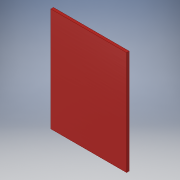
# Autodesk Inventor part: GBX_001.1-side-plate
Saved by Autodesk Inventor 2019 (Build 230136000, 136)
## iProperties
Created: 2019-08-15
Part Number: GBX_001.1-side-plate
Material: Generic
Document SubType Name: Modeling
Designer: Rene
Density: 1 g/cm^3
Appearance: Orange-Red
Author: Rene
Autodesk Inventor part; units mm, degrees
ref_plane "YZ Plane" through (0, 0, 0) normal (1, 0, 0) x (0, 1, 0)
ref_plane "XZ Plane" through (0, 0, 0) normal (0, 1, 0) x (-1, 0, 0)
ref_plane "XY Plane" through (0, 0, 0) normal (0, 0, 1) x (1, 0, 0)
sketch "Sketch1" plane through (0, 0, 0) normal (0, 0, 1) x (1, 0, 0)
  line L0 (175, -240) -> (-175, -240)
  line L1 (-175, -240) -> (-175, 240)
  line L2 (-175, 240) -> (175, 240)
  line L3 (175, 240) -> (175, -240)
  line L4 (175, -240) -> (-175, 240) construction
  line L5 (-175, -240) -> (175, 240) construction
  point P0 (0, 0)
  dimension "d0" = 480
  dimension "d1" = 350
  constraints: 12 end point, 2 midpoint, 2 parallel, 1 horizontal, 1 perpendicular
  measures "d0" distance of L0.end L1.end
  measures "d1" distance of L1.end L2.end
extrude "Extrusion1" add sketch "Sketch1" along normal blind 12
body "Solid1"
